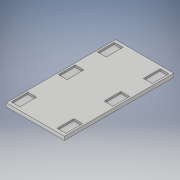
# Autodesk Inventor part: BODY_BOTTOM
Saved by Autodesk Inventor 2017 (Build 210142000, 142)
## iProperties
Created: 2017-08-24
Part Number: BODY_BOTTOM
Material: Generic
Document SubType Name: Modeling
Designer: Alexander Miller
Density: 1 g/cm^3
Appearance: Default
body_A: 150,000 mm
body_B: 80,000 mm
body_C: 5,000 mm
Author: Alexander Miller
Autodesk Inventor part; units mm, degrees
ref_plane "YZ Plane" through (0, 0, 0) normal (1, 0, 0) x (0, 1, 0)
ref_plane "XZ Plane" through (0, 0, 0) normal (0, 1, 0) x (-1, 0, 0)
ref_plane "XY Plane" through (0, 0, 0) normal (0, 0, 1) x (1, 0, 0)
sketch "Sketch4" plane through (0, 0, 0) normal (0, 1, 0) x (-1, 0, 0)
  line L0 (40, 75) -> (-40, 75)
  line L1 (-40, 75) -> (-40, -75)
  line L2 (-40, -75) -> (40, -75)
  line L3 (40, -75) -> (40, 75)
  point P0 (0, 0)
  point P1 (0, -75)
  point P2 (40, 0)
  dimension "d15" = 150
  dimension "d16" = 80
  constraints: 8 end point, 2 midpoint, 2 parallel, 1 horizontal, 1 horizontal alignment, 1 perpendicular, 1 vertical alignment
  measures "d15" distance of L2.end L0.start
  measures "d16" distance of L1.end L2.end
extrude "Extrusion3" add sketch "Sketch4" along normal blind 5
sketch "Sketch5" plane through (0, 5, 0) normal (0, 1, 0) x (1, 0, 0)
  line L0 (-37.5, 70.75) -> (-25.5, 70.75)
  line L1 (-25.5, 70.75) -> (-25.5, 47.75)
  line L2 (-25.5, 47.75) -> (-37.5, 47.75)
  line L3 (-37.5, 47.75) -> (-37.5, 70.75)
  line L4 (-37.5, 17) -> (-25.5, 17)
  line L5 (-25.5, 17) -> (-25.5, -6)
  line L6 (-25.5, -6) -> (-37.5, -6)
  line L7 (-37.5, -6) -> (-37.5, 17)
  line L8 (-37.5, -47.75) -> (-25.5, -47.75)
  line L9 (-25.5, -47.75) -> (-25.5, -70.75)
  line L10 (-25.5, -70.75) -> (-37.5, -70.75)
  line L11 (-37.5, -70.75) -> (-37.5, -47.75)
  line L12 (40, 75) -> (-40, 75) projected
  line L13 (-40, 75) -> (-40, -75) projected
  line L14 (-40, -75) -> (40, -75) projected
  circle A0 centre (-31.5, 0) radius 6 construction
  line L15 (0, 105) -> (0, -105) construction
  line L16 (37.5, 70.75) -> (25.5, 70.75)
  line L17 (25.5, 70.75) -> (25.5, 47.75)
  line L18 (25.5, 47.75) -> (37.5, 47.75)
  line L19 (37.5, 47.75) -> (37.5, 70.75)
  line L20 (37.5, 17) -> (25.5, 17)
  line L21 (25.5, 17) -> (25.5, -6)
  line L22 (25.5, -6) -> (37.5, -6)
  line L23 (37.5, -6) -> (37.5, 17)
  line L24 (37.5, -47.75) -> (25.5, -47.75)
  line L25 (25.5, -47.75) -> (25.5, -70.75)
  line L26 (25.5, -70.75) -> (37.5, -70.75)
  line L27 (37.5, -70.75) -> (37.5, -47.75)
  point P0 (0, 0)
  point P1 (-31.5, 47.75)
  point P2 (-31.5, 17)
  point P3 (-31.5, -6)
  point P4 (-31.5, -47.75)
  dimension "d19" = 23
  dimension "d20" = 12
  dimension "d21" = 4.25
  dimension "d22" = 2.5
  dimension "d23" = 4.25
  constraints: 48 end point, 12 symmetric about line, 6 parallel, 4 equal length, 4 midpoint, 3 horizontal, 3 perpendicular, 3 tangent, 2 vertical alignment, 1 centre point, 1 horizontal alignment
  measures "d19" distance of L2.end L0.start
  measures "d20" distance of L0.start L0.end
  measures "d21" distance between parallel lines of L0 L12
  measures "d22" distance between parallel lines of L3 L13
  measures "d23" distance between parallel lines of L14 L10
extrude "Extrusion4" cut sketch "Sketch5" against normal blind 2.5
equation "\"d15\" = body_A"
equation "\"d16\" = body_B"
equation "\"d17\" = body_C"
equation "\"d19\" = servo_A"
equation "\"d20\" = servo_B"
equation "\"d21\" = -0.5 * servo_A + 0.5 * servo_D"
equation "\"d22\" = 0.5 * body_C"
equation "\"d23\" = d21"
equation "\"d26\" = 0.5 * body_C"
equation "\"body_A\" = 150"
equation "\"body_B\" = 80"
equation "\"body_C\" = 5"
equation "\"body_D\" = 0.25 * servo_D"
equation "\"body_E\" = 0.25 * servo_D"
equation "\"servo_A\" = 23"
equation "\"servo_B\" = 12"
equation "\"servo_D\" = 31.5"
body "Solid2"
